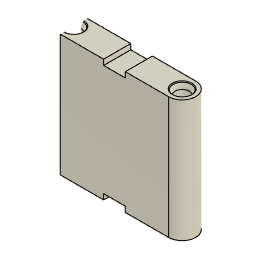
Tool_Dowel_Fixture-Parametric (Autodesk Fusion 360 design; units mm, degrees)
Autodesk Fusion 360 part; units mm, degrees
sketch "Sketch1" plane through (0, 0, 0) normal (0, 0, 1) x (1, 0, 0)
  circle A0 centre (0, 0) radius 2.65
  circle A1 centre (0, 0) radius 5
  line L0 (0, 0) -> (40, 0) construction
  circle A2 centre (40, 0) radius 2.65
  circle A3 centre (40, 0) radius 5
  line L1 (0, -5) -> (40, -5)
  line L2 (0, 5) -> (40, 5)
  dimension "d3" = 5.3
  dimension "d4" = 10
  dimension "d5" = 40
  dimension "d6" = 5.3
  dimension "d7" = 10
  constraint coincident A0.centre A1.centre
  constraint concentric A0 A1
  constraint horizontal L0
  constraint coincident L0.end A2.centre
  constraint concentric A2 A3
  constraint coincident A1 L1.start
  constraint coincident A3 L1.end
  constraint tangent A3 L1
  constraint horizontal L1
  constraint coincident A1 L2.start
  constraint coincident A3 L2.end
  constraint tangent A3 L2
  constraint parallel L1 L2
  measures "d3" diameter of A0
  measures "d4" diameter of A1
  measures "d5" distance of A0.centre L0.end
  measures "d6" diameter of A2
  measures "d7" diameter of A3
extrude "Extrude1" add sketch "Sketch1" along normal blind 45
chamfer "Chamfer1" distance 1 angle 45 2 edges at (-2.4707, 0.9583, 45) (37.5293, 0.9583, 45)
fillet "Fillet1" radius 2.5 2 edges at (-2.4707, 0.9583, 44) (37.5293, 0.9583, 44)
ref_plane "WorkPlane1" through (0, 0, 0) normal (1, 0, 0) x (0, 1, 0)
chamfer "Chamfer2" distance 1 angle 45 2 edges at (-2.4707, 0.9583, 0) (37.5293, 0.9583, 0)
sketch "Sketch2" plane through (0, -5, 0) normal (0, -1, 0) x (1, 0, 0)
  line L0 (0, 0) -> (40, 0)
  line L1 (40, 0) -> (40, 45)
  line L2 (40, 45) -> (0, 45)
  line L3 (0, 45) -> (0, 0)
  line L4 (20, 45) -> (20, 43)
  line L5 (20, 43) -> (16, 43)
  line L6 (16, 43) -> (16, 45)
  line L7 (16, 45) -> (20, 45)
  line L8 (20, 45) -> (20, 43)
  line L9 (20, 45) -> (24, 45)
  line L10 (24, 45) -> (24, 43)
  line L11 (24, 43) -> (20, 43)
  line L12 (20, 43) -> (20, 45)
  line L13 (20, 0) -> (16, 0)
  line L14 (16, 0) -> (16, 2)
  line L15 (16, 2) -> (20, 2)
  line L16 (20, 2) -> (20, 0)
  line L17 (20, 0) -> (24, 0)
  line L18 (24, 0) -> (24, 2)
  line L19 (24, 2) -> (20, 2)
  line L20 (20, 2) -> (20, 0)
  dimension "d15" = 2
  dimension "d16" = 4
  dimension "d17" = 4
  dimension "d18" = 4
  dimension "d19" = 2
  dimension "d20" = 4
  dimension "d21" = 2
  constraint midpoint L2 L4.start
  constraint perpendicular L2 L4
  constraint horizontal L5
  constraint vertical L6
  constraint horizontal L7
  constraint vertical L8
  constraint horizontal L9
  constraint vertical L10
  constraint horizontal L11
  constraint vertical L12
  constraint horizontal L13
  constraint vertical L14
  constraint horizontal L15
  constraint vertical L16
  constraint midpoint L0 L13.start
  constraint horizontal L17
  constraint vertical L18
  constraint horizontal L19
  constraint vertical L20
  measures "d15" distance of L4.start L4.end
  measures "d16" distance of L4.end L5.end
  measures "d17" distance of L4.start L9.end
  measures "d18" distance of L13.start L13.end
  measures "d19" distance of L13.start L15.end
  measures "d20" distance of L13.start L17.end
  measures "d21" distance of L13.start L15.end
extrude "Extrude2" cut sketch "Sketch2" against normal blind 14 contours L0 L13 L14 L15 L16 L20 | L0 L16 L17 L18 L19 L20 | L2 L4 L5 L6 L7 L8 L12 | L2 L4 L8 L9 L10 L11 L12
fillet "Fillet2" radius 2.5 2 edges at (-2.4707, -0.9583, 1) (37.5293, -0.9583, 1)
equation "spacing = 40 mm" comment "babyBullet=40mm"
equation "holeSize = 5.30 mm" comment "resize for tollerance"
equation "d3 = holeSize"
equation "d5 = spacing"
equation "d6 = holeSize"
